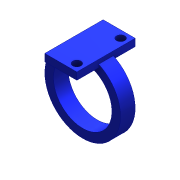
# Autodesk Inventor part: Ring
Saved by Autodesk Inventor 2016 (Build 200138000, 138)
## iProperties
Created: 2017-09-09
Part Number: Ring
Material: Generic
Document SubType Name: Modeling
Designer: rishi
Density: 1 g/cm^3
Appearance: Blue - Wall Paint - Glossy
Author: rishi
Autodesk Inventor part; units mm, degrees
ref_plane "YZ Plane" through (0, 0, 0) normal (1, 0, 0) x (0, 1, 0)
ref_plane "XZ Plane" through (0, 0, 0) normal (0, 1, 0) x (-1, 0, 0)
sketch "Sketch2" plane through (0, 0, 0) normal (0, 1, 0) x (-1, 0, 0)
  circle A0 centre (0, 0) radius 10
  circle A1 centre (0, 0) radius 13
  dimension "d7" = 20
  dimension "d8" = 26
  constraints: 2 centre point, 2 coincident
  measures "d7" diameter of A0
  measures "d8" diameter of A1
extrude "Extrusion1" add sketch "Sketch2" along normal blind 5
sketch "Sketch3" plane through (0, 0, 0) normal (0, 0, 1) x (1, 0, 0)
  point P0 (0, 0)
ref_plane "Work Plane1" through (0, 0, 12) normal (0, 0, 1) x (1, 0, 0)
sketch "Sketch4" plane through (0, 0, 12) normal (0, 0, 1) x (1, 0, 0)
  point P0 (0, 0)
sketch "Sketch5" plane through (0, 0, 12) normal (0, 0, 1) x (1, 0, 0)
  line L0 (-13, 0) -> (13, 0) projected
  line L1 (5.5, 0) -> (-5.5, 0)
  line L2 (-5.5, 0) -> (-5.5, 12.5)
  line L3 (-5.5, 12.5) -> (5.5, 12.5)
  line L4 (5.5, 12.5) -> (5.5, 0)
  line L5 (-5.5, 0) -> (5.5, 0)
  line L6 (5.5, 0) -> (5.5, -7.5)
  line L7 (5.5, -7.5) -> (-5.5, -7.5)
  line L8 (-5.5, -7.5) -> (-5.5, 0)
  line L9 (0, -16.9) -> (0, 20.9) projected
  dimension "d16" = 11
  dimension "d17" = 7.5
  dimension "d18" = 12.5
  dimension "d19" = 5.5
  constraints: 16 end point, 4 parallel, 2 horizontal, 2 perpendicular, 2 point on line
  measures "d16" distance of L2.end L3.end
  measures "d17" distance of L5.end L6.end
  measures "d18" distance of L3.end L1.start
  measures "d19" distance between parallel lines of L4 L9
extrude "Extrusion2" add sketch "Sketch5" along normal mid plane 2.5
sketch "Sketch6" plane through (0, 0, 13.25) normal (0, 0, 1) x (1, 0, 0)
  line L0 (5.5, -7.5) -> (5.5, 12.5) projected
  line L1 (5.5, 12.5) -> (-5.5, 12.5) projected
  line L2 (-5.5, -7.5) -> (5.5, -7.5) projected
  point P0 (0, 0)
  point P1 (3, 10)
  point P2 (3, -5)
  dimension "d20" = 2.5
  dimension "d21" = 2.5
  dimension "d22" = 2.5
  dimension "d30" = 2.5
  measures "d20" distance from line of L0 point (3, 10)
  measures "d21" distance from line of L1 point (3, 10)
  measures "d22" distance from line of L2 point (3, -5)
  measures "d30" distance from line of L0 point (3, -5)
hole "Hole1" at (3, -5, 13.25) at (3, 10, 13.25) direction (0, 0, -1) diameter 2.85 depth 8 tip angle 118
body "Solid1"
